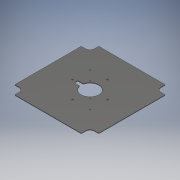
# Autodesk Inventor part: -ZPanel_PCB
Saved by Autodesk Inventor 2018 (Build 220112000, 112)
## iProperties
Created: 2018-11-03
Part Number: -ZPanel_PCB
Material: Epoxy Resin
Document SubType Name: Modeling
Designer: Bradley
Density: 1.14 g/cm^3
Appearance: Smooth - Dark Gray
Mass: 5.79181 g
Surface Area: 172.339 cm^2
Volume: 5.08053 cm^3
Author: Bradley
Autodesk Inventor part; units mm, degrees
ref_plane "YZ Plane" through (0, 0, 0) normal (1, 0, 0) x (0, 1, 0)
ref_plane "XZ Plane" through (0, 0, 0) normal (0, 1, 0) x (-1, 0, 0)
ref_plane "XY Plane" through (0, 0, 0) normal (0, 0, 1) x (1, 0, 0)
sketch "Sketch1" plane through (0, 0, 0) normal (0, 0, 1) x (1, 0, 0)
  line L0 (-48, -48) -> (48, -48)
  line L1 (48, -48) -> (48, 48)
  line L2 (48, 48) -> (-48, 48)
  line L3 (-48, 48) -> (-48, -48)
  line L4 (-48, -48) -> (48, 48) construction
  line L5 (48, -48) -> (-48, 48) construction
  line L6 (-38, 48) -> (-38, 43)
  arc A0 (-43, 38) -> (-38, 43) centre (-43, 43) ccw
  line L7 (-43, 38) -> (-48, 38)
  circle A1 centre (0, 0) radius 40 construction
  line L8 (38, 48) -> (38, 43)
  arc A2 (38, 43) -> (43, 38) centre (43, 43) ccw
  line L9 (43, 38) -> (48, 38)
  line L10 (48, -38) -> (43, -38)
  arc A3 (43, -38) -> (38, -43) centre (43, -43) ccw
  line L11 (38, -43) -> (38, -48)
  line L12 (-38, -48) -> (-38, -43)
  arc A4 (-38, -43) -> (-43, -38) centre (-43, -43) ccw
  line L13 (-43, -38) -> (-48, -38)
  circle A5 centre (0, 0) radius 10
  line L14 (-9.798, 2) -> (-15, 2)
  arc A6 (-15, 2) -> (-16, 1) centre (-15, 1) ccw
  line L15 (-16, 1) -> (-16, -1)
  arc A7 (-16, -1) -> (-15, -2) centre (-15, -1) ccw
  line L16 (-15, -2) -> (-9.798, -2)
  dimension "d0" = 96
  dimension "d1" = 96
  dimension "d2" = 10
  dimension "d3" = 80
  dimension "d4" = 5
  dimension "d7" = 20
  dimension "d8" = 1
  dimension "d9" = 4
  dimension "d10" = 16
  constraints: 34 end point, 14 point on circle, 11 point on line, 11 tangent, 8 centre point, 7 equal length, 6 perpendicular, 4 equal radius, 3 horizontal, 3 vertical, 2 coincident, 2 midpoint, 2 parallel
  measures "d0" distance of L2.end L1.end
  measures "d1" distance of L1.end L0.end
  measures "d2" distance between parallel lines of L2 L7
  measures "d3" diameter of A1
  measures "d4" radius of A0
  measures "d7" diameter of A5
  measures "d8" radius of A6
  measures "d9" distance between parallel lines of L16 L14
  measures "d10" distance from line of point (0, 0) L15
extrude "Extrusion1" add sketch "Sketch1" along normal mid plane 0.6 contours L12 A4 L13 L3 L7 A0 L6 L2 L8 A2 L9 L1 L10 A3 L11 L0
fillet "Fillet1" radius 0.5 10 edges at (-9.798, 2, 0) (-9.798, -2, 0) (-38, 48, 0) (-48, 38, 0) (38, 48, 0) (48, 38, 0) (48, -38, 0) (38, -48, 0) (-38, -48, 0) (-48, -38, 0)
sketch "Sketch2" plane through (0, 0, 0.3) normal (0, 0, 1) x (1, 0, 0)
  line L0 (19.4454, -19.4454) -> (8.8388, -8.8388) construction
  line L1 (-19.4454, 19.4454) -> (-8.8388, 8.8388) construction
  arc A0 (-48, -37.5) -> (-47.5, -38) centre (-47.5, -37.5) ccw projected
  line L2 (-47.5, -38) -> (-43, -38) projected
  arc A1 (-38, -43) -> (-43, -38) centre (-43, -43) ccw projected
  line L3 (-38, -43) -> (-38, -47.5) projected
  arc A2 (-38, -47.5) -> (-37.5, -48) centre (-37.5, -47.5) ccw projected
  line L4 (-37.5, -48) -> (37.5, -48) projected
  arc A3 (37.5, -48) -> (38, -47.5) centre (37.5, -47.5) ccw projected
  line L5 (38, -47.5) -> (38, -43) projected
  arc A4 (43, -38) -> (38, -43) centre (43, -43) ccw projected
  line L6 (43, -38) -> (47.5, -38) projected
  arc A5 (47.5, -38) -> (48, -37.5) centre (47.5, -37.5) ccw projected
  line L7 (48, -37.5) -> (48, 37.5) projected
  arc A6 (48, 37.5) -> (47.5, 38) centre (47.5, 37.5) ccw projected
  line L8 (47.5, 38) -> (43, 38) projected
  arc A7 (38, 43) -> (43, 38) centre (43, 43) ccw projected
  line L9 (38, 43) -> (38, 47.5) projected
  arc A8 (38, 47.5) -> (37.5, 48) centre (37.5, 47.5) ccw projected
  line L10 (37.5, 48) -> (-37.5, 48) projected
  arc A9 (-37.5, 48) -> (-38, 47.5) centre (-37.5, 47.5) ccw projected
  line L11 (-38, 47.5) -> (-38, 43) projected
  arc A10 (-43, 38) -> (-38, 43) centre (-43, 43) ccw projected
  line L12 (-43, 38) -> (-47.5, 38) projected
  arc A11 (-47.5, 38) -> (-48, 37.5) centre (-47.5, 37.5) ccw projected
  line L13 (-48, 37.5) -> (-48, -37.5) projected
  arc A12 (-9.7124, -2.381) -> (-10.198, -2) centre (-10.198, -2.5) ccw projected
  line L14 (-10.198, -2) -> (-15, -2) projected
  arc A13 (-16, -1) -> (-15, -2) centre (-15, -1) ccw projected
  line L15 (-16, -1) -> (-16, 1) projected
  arc A14 (-15, 2) -> (-16, 1) centre (-15, 1) ccw projected
  line L16 (-15, 2) -> (-10.198, 2) projected
  arc A15 (-10.198, 2) -> (-9.7124, 2.381) centre (-10.198, 2.5) ccw projected
  arc A16 (-9.7124, -2.381) -> (-9.7124, 2.381) centre (0, 0) ccw projected
  circle A17 centre (0, 0) radius 12.5 construction
  dimension "d12" = 15
  dimension "d33" = 135
  dimension "d34" = 25
  constraints: 5 coincident, 4 end point, 2 collinear, 2 point on circle, 1 centre point, 1 point on line
  measures "d12" distance of L1.start L1.end
  measures "d33" angle of L4 L1
  measures "d34" diameter of A17
hole "Hole1" at (-8.8388, 8.8388, 0.3) at (-19.4454, 19.4454, 0.3) at (8.8388, -8.8388, 0.3) at (19.4454, -19.4454, 0.3) direction (0, 0, -1) diameter 1 end through all
sketch "Sketch3" plane through (0, 0, 0.3) normal (0, 0, 1) x (1, 0, 0)
  point P0 (0, 0)
  point P1 (-20, 0)
  point P2 (0, -20)
  point P3 (20, 0)
  point P4 (0, 20)
  dimension "d21" = 20
  dimension "d24" = 360
  constraints: 1 horizontal alignment, 5 other
  measures "d21" distance of point (-20, 0) point (0, 0)
hole "Hole2" at (-20, 0, 0.3) at (0, -20, 0.3) at (20, 0, 0.3) at (0, 20, 0.3) direction (0, 0, -1) diameter 1.6 end through all
body "Solid1"
